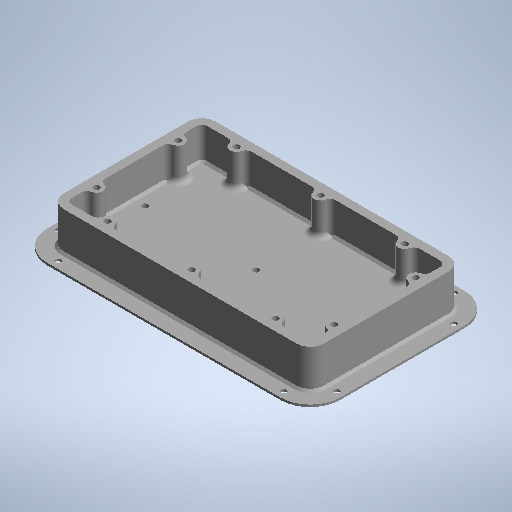
# Autodesk Inventor part: RT_ELE_MC_020_ExtPowerFilterCaseBottom
Saved by Autodesk Inventor 2025.4 (Build 294407000, 407)
## iProperties
Created: 2026-08-13
Part Number: RT_ELE_MC_020_ExtPowerFilterCaseBottom
Material: Générique
Document SubType Name: Modeling
Designer: louis
Density: 1 g/cm^3
Appearance: Par défaut
Author: louis
Autodesk Inventor part; units mm, degrees
ref_plane "YZ Plane" through (0, 0, 0) normal (1, 0, 0) x (0, 1, 0)
ref_plane "XZ Plane" through (0, 0, 0) normal (0, 1, 0) x (-1, 0, 0)
ref_plane "XY Plane" through (0, 0, 0) normal (0, 0, 1) x (1, 0, 0)
sketch "Sketch2" plane through (0, 0, 0) normal (0, 0, 1) x (1, 0, 0)
  line L0 (-120, -70) -> (120, -70)
  line L1 (120, -70) -> (120, 70)
  line L2 (120, 70) -> (-120, 70)
  line L3 (-120, 70) -> (-120, -70)
  line L4 (-120, -70) -> (120, 70) construction
  line L5 (120, -70) -> (-120, 70) construction
  line L6 (-112.5, 62.5) -> (112.5, 62.5)
  line L7 (112.5, 62.5) -> (112.5, -62.5)
  line L8 (112.5, -62.5) -> (-112.5, -62.5)
  line L9 (-112.5, -62.5) -> (-112.5, 62.5)
  line L10 (-110, -17.5) -> (110, -17.5) construction
  line L11 (110, -17.5) -> (110, 17.5) construction
  line L12 (110, 17.5) -> (-110, 17.5) construction
  line L13 (-110, 17.5) -> (-110, -17.5) construction
  line L14 (-110, -17.5) -> (110, 17.5) construction
  line L15 (110, -17.5) -> (-110, 17.5) construction
  line L16 (-10, 50) -> (100, 50) construction
  line L17 (100, 50) -> (100, -50) construction
  line L18 (100, -50) -> (-10, -50) construction
  line L19 (-10, -50) -> (-10, 50) construction
  line L20 (-10, 50) -> (100, -50) construction
  line L21 (-10, -50) -> (100, 50) construction
  line L22 (0, 0) -> (110, 0) construction
  circle A0 centre (-109.5, 37.5) radius 2.8
  circle A1 centre (77.5, 59.5) radius 2.8
  circle A2 centre (-77.5, 59.5) radius 2.8
  circle A3 centre (-109.5, -37.5) radius 2.8
  circle A4 centre (-77.5, -59.5) radius 2.8
  circle A5 centre (109.5, 37.5) radius 2.8
  circle A6 centre (109.5, -37.5) radius 2.8
  circle A7 centre (77.5, -59.5) radius 2.8
  line L23 (0, 0) -> (0, 62.5) construction
  circle A8 centre (0, 59.5) radius 2.8
  circle A9 centre (0, -59.5) radius 2.8
  circle A10 centre (-77.5, 59.5) radius 6
  circle A11 centre (77.5, 59.5) radius 6
  circle A12 centre (0, 59.5) radius 6
  circle A13 centre (-109.5, 37.5) radius 6
  circle A14 centre (109.5, 37.5) radius 6
  circle A15 centre (-77.5, -59.5) radius 6
  circle A16 centre (77.5, -59.5) radius 6
  circle A17 centre (0, -59.5) radius 6
  circle A18 centre (-109.5, -37.5) radius 6
  circle A19 centre (109.5, -37.5) radius 6
  point P0 (100, 0)
  point P1 (-112.5, -32.3038)
  point P2 (-112.5, -42.6962)
  point P3 (-82.6962, -62.5)
  point P4 (-72.3038, -62.5)
  point P5 (-5.1962, -62.5)
  point P6 (5.1962, -62.5)
  point P7 (72.3038, -62.5)
  point P8 (82.6962, -62.5)
  point P9 (112.5, -42.6962)
  point P10 (112.5, -32.3038)
  point P11 (112.5, 32.3038)
  point P12 (112.5, 42.6962)
  point P13 (72.3038, 62.5)
  point P14 (82.6962, 62.5)
  point P15 (-5.1962, 62.5)
  point P16 (5.1962, 62.5)
  point P17 (-82.6962, 62.5)
  point P18 (-72.3038, 62.5)
  point P19 (-112.5, 42.6962)
  point P20 (-112.5, 32.3038)
  dimension "d0" = 240
  dimension "d1" = 140
  dimension "d2" = 7.5
  dimension "d7" = 220
  dimension "d8" = 35
  dimension "d9" = 110
  dimension "d10" = 100
  dimension "d11" = 10
  dimension "d14" = 5.6
  dimension "d16" = 5.6
  dimension "d22" = 3
  dimension "d23" = 3
  dimension "d24" = 5.6
  dimension "d26" = 3
  dimension "d27" = 25
  dimension "d28" = 35
  dimension "d30" = 12
  dimension "d31" = 12
  dimension "d32" = 12
  dimension "d33" = 12
  dimension "d34" = 12
  constraints: 48 end point, 20 centre point, 8 parallel, 7 midpoint, 5 symmetric about line, 4 coincident, 4 perpendicular, 3 horizontal, 2 point on line, 15 other
  measures "d0" distance of L2.end L1.end
  measures "d1" distance of L1.end L0.end
  measures "d2" distance between parallel lines of L2 L6
  measures "d7" distance of L12.end L11.end
  measures "d8" distance of L11.end L10.end
  measures "d9" distance of L17.end L18.end
  measures "d10" distance of L16.end L17.end
  measures "d11" distance from line of point (100, 0) L11
  measures "d14" diameter of A0
  measures "d16" diameter of A2
  measures "d22" distance from line of L6 A2.centre
  measures "d23" distance from line of L9 A0.centre
  measures "d24" diameter of A8
  measures "d26" distance from line of L6 A8.centre
  measures "d27" distance from line of L6 A0.centre
  measures "d28" distance from line of L9 A2.centre
  measures "d30" diameter of A13
  measures "d31" diameter of A10
  measures "d32" diameter of A11
  measures "d33" diameter of A12
  measures "d34" diameter of A14
extrude "Extrusion1" add sketch "Sketch2" along normal blind 30 contours L3 L2 L1 L0 | A10 L6 | L9 A13 | A12 L6 | L9 A18 | A11 L6 | L8 A15 | A14 L7 | L8 A17 | A19 L7 | L8 A16 picked at (-77.7322, 63.4865) picked at (-112.8725, 36.0453) picked at (0.684, 63.3794) picked at (-112.8725, -38.9547) picked at (77.2678, 63.4865) picked at (-77.0992, -64.1575) picked at (112.8383, 36.0137) picked at (-1.4547, -62.8725) picked at (112.8383, -38.9863) picked at (77.9008, -64.1575)
extrude "Extrusion2" add sketch "Sketch2" against normal blind 7.5 contours L3 L2 L1 L0 | L6 A10 A12 A11 L7 A14 A19 L8 A16 A17 A15 L9 A18 A13 | A10 L6 | L6 A10 | A13 L9 | L9 A13 | A12 L6 | L6 A12 | A18 L9 | L9 A18 | A11 L6 | L6 A11 | A15 L8 | L8 A15 | A14 L7 | L7 A14 | A17 L8 | L8 A17 | A19 L7 | L7 A19 | A16 L8 | L8 A16 | A0 | A1 | A2 | A3 | A4 | A5 | A6 | A7 | A8 | A9
fillet "Fillet1" radius 5 4 edges at (-112.5, 62.5, 15) (-112.5, -62.5, 15) (112.5, -62.5, 15) (112.5, 62.5, 15)
fillet "Fillet2" radius 12.5 4 edges at (-120, 70, 11.25) (-120, -70, 11.25) (120, -70, 11.25) (120, 70, 11.25)
chamfer "Chamfer1" distance 2 angle 45 16 edges at (0, -62.5, 0) (-111.0355, -61.0355, 0) (-112.5, 0, 0) (-111.0355, 61.0355, 0) (0, 62.5, 0) (111.0355, 61.0355, 0) (112.5, 0, 0) (111.0355, -61.0355, 0) (0, -70, -7.5) (-116.3388, -66.3388, -7.5) (-120, 0, -7.5) (-116.3388, 66.3388, -7.5) (0, 70, -7.5) (116.3388, 66.3388, -7.5) (120, 0, -7.5) (116.3388, -66.3388, -7.5)
extrude "Extrusion3" add sketch "Sketch2" along normal blind 30 contours L6 A10 | A13 L9 | L6 A12 | A18 L9 | L6 A11 | A15 L8 | L7 A14 | A17 L8 | L7 A19 | A16 L8 picked at (-72.6532, 58.7928) picked at (-104.6206, 37.9612) picked at (4.8468, 58.7928) picked at (-104.6206, -37.0388) picked at (82.3468, 58.7928) picked at (-72.6532, -58.7928) picked at (111.3783, 42.0284) picked at (4.8468, -58.7928) picked at (111.3783, -42.0284) picked at (82.3468, -58.7928)
fillet "Fillet3" radius 5 30 edges at (-5.1962, 62.5, 16) (5.1962, 62.5, 16) (-82.6962, 62.5, 16) (-72.3038, 62.5, 16) (-112.5, 32.3038, 16) (-112.5, 42.6962, 16) (-112.5, -42.6962, 16) (-112.5, -32.3038, 16) (-72.3038, -62.5, 16) (-82.6962, -62.5, 16) (82.6962, -62.5, 16) (72.3038, -62.5, 16) (5.1962, -62.5, 16) (-5.1962, -62.5, 16) (112.5, -32.3038, 16) (112.5, -42.6962, 16) (112.5, 42.6962, 16) (112.5, 32.3038, 16) (72.3038, 62.5, 16) (82.6962, 62.5, 16) (-103.5, 37.5, 0) (-77.5, 53.5, 0) (0, 53.5, 0) (77.5, 53.5, 0) (103.5, 37.5, 0) (103.5, -37.5, 0) (77.5, -53.5, 0) (0, -53.5, 0) (-77.5, -53.5, 0) (-103.5, -37.5, 0)
sketch "Sketch3" plane through (0, 0, -7.5) normal (0, 0, -1) x (-1, 0, 0)
  line L0 (107.5, -68) -> (-107.5, -68) projected
  arc A0 (107.5, -68) -> (118, -57.5) centre (107.5, -57.5) ccw projected
  line L1 (118, 57.5) -> (118, -57.5) projected
  arc A1 (118, 57.5) -> (107.5, 68) centre (107.5, 57.5) ccw projected
  line L2 (-107.5, 68) -> (107.5, 68) projected
  arc A2 (-107.5, 68) -> (-118, 57.5) centre (-107.5, 57.5) ccw projected
  line L3 (-118, -57.5) -> (-118, 57.5) projected
  arc A3 (-118, -57.5) -> (-107.5, -68) centre (-107.5, -57.5) ccw projected
  arc A4 (135, 57.5) -> (107.5, 85) centre (107.5, 57.5) ccw
  line L4 (135, 57.5) -> (135, -57.5)
  arc A5 (107.5, -85) -> (135, -57.5) centre (107.5, -57.5) ccw
  line L5 (107.5, -85) -> (-107.5, -85)
  arc A6 (-135, -57.5) -> (-107.5, -85) centre (-107.5, -57.5) ccw
  line L6 (-135, -57.5) -> (-135, 57.5)
  arc A7 (-107.5, 85) -> (-135, 57.5) centre (-107.5, 57.5) ccw
  line L7 (-107.5, 85) -> (107.5, 85)
  point P0 (0, 0)
  dimension "d41" = 17
  constraints: 8 end point, 8 point on circle, 4 centre point, 7 other
  measures "d41" distance between parallel lines of L2 L7
extrude "Extrusion4" add sketch "Sketch3" against normal blind 2
chamfer "Chamfer2" distance 2 angle 45 8 edges at (120, 0, -5.5) (116.3388, -66.3388, -5.5) (0, -70, -5.5) (-116.3388, -66.3388, -5.5) (-120, 0, -5.5) (-116.3388, 66.3388, -5.5) (0, 70, -5.5) (116.3388, 66.3388, -5.5)
sketch "Sketch4" plane through (0, 0, -5.5) normal (0, 0, 1) x (1, 0, 0)
  circle A0 centre (104, -78.5) radius 2.55
  circle A1 centre (128.5, -54) radius 2.55
  line L0 (110.5, -48.4545) -> (110.5, -57.5) projected
  line L1 (-107.5, -72) -> (107.5, -72) projected
  line L2 (-107.5, -85) -> (107.5, -85) projected
  line L3 (122, -57.5) -> (122, 57.5) projected
  line L4 (107.5, -60.5) -> (88.4545, -60.5) projected
  point P0 (0, 0)
  point P1 (110.5, -52.9772)
  dimension "d47" = 5.1
  dimension "d48" = 5.1
  dimension "d50" = 6.5
  dimension "d52" = 6.5
  dimension "d53" = 6.5
  dimension "d54" = 6.5
  constraints: 2 centre point, 1 midpoint
  measures "d47" diameter of A0
  measures "d48" diameter of A1
  measures "d50" distance from line of L1 A0.centre
  measures "d52" distance from line of L3 A1.centre
  measures "d53" distance from line of L4 A1.centre
  measures "d54" distance from line of L0 A0.centre
extrude "Extrusion5" cut sketch "Sketch4" against normal through all
mirror "Mirror1" about plane through (0, 0, 0) normal (0, 1, 0) of "Extrusion5"
mirror "Mirror2" about plane through (0, 0, 0) normal (1, 0, 0) of "Extrusion5", "Mirror1"
sketch "Sketch5" plane through (0, 0, 0) normal (0, 0, 1) x (1, 0, 0)
  line L0 (-110, 0) -> (110, 0) construction
  circle A0 centre (100, 0) radius 2.8
  circle A1 centre (-102.5, 0) radius 2.8
  circle A2 centre (0, 0) radius 2.8
  line L1 (-112.5, -26.6833) -> (-112.5, 26.6833) projected
  point P0 (-112.5, 0)
  dimension "d57" = 220
  dimension "d58" = 5.6
  dimension "d59" = 5.6
  dimension "d60" = 5.6
  dimension "d61" = 10
  dimension "d62" = 10
  constraints: 3 centre point, 2 end point, 2 midpoint, 2 point on line, 1 coincident, 1 horizontal
  measures "d57" distance of L0.start L0.end
  measures "d58" diameter of A0
  measures "d59" diameter of A1
  measures "d60" diameter of A2
  measures "d61" distance of L0.end A0.centre
  measures "d62" distance of point (-112.5, 0) A1.centre
extrude "Extrusion6" cut sketch "Sketch5" against normal through all
equation "\"d30\" = d31"
equation "\"d32\" = d31"
equation "\"d33\" = d31"
equation "\"d34\" = d31"
body "Solid1"
